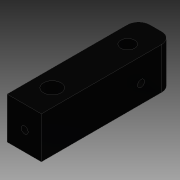
# Autodesk Inventor part: Fixture_Base
Saved by Autodesk Inventor 2015 SP1 (Build 190203100, 203)
## iProperties
Created: 2014-12-16
Part Number: Fixture_Base
Material: Generic
Document SubType Name: Modeling
Designer: amarschn
Density: 1 g/cm^3
Appearance: Anodized - Black
Author: amarschn
Autodesk Inventor part; units mm, degrees
ref_plane "YZ Plane" through (0, 0, 0) normal (1, 0, 0) x (0, 1, 0)
ref_plane "XZ Plane" through (0, 0, 0) normal (0, 1, 0) x (-1, 0, 0)
ref_plane "XY Plane" through (0, 0, 0) normal (0, 0, 1) x (1, 0, 0)
sketch "Sketch1" plane through (0, 0, 0) normal (0, 1, 0) x (-1, 0, 0)
  line L0 (-5.3975, -59.69) -> (5.3975, -59.69)
  line L1 (15.5575, -49.53) -> (15.5575, 59.69)
  line L2 (15.5575, 59.69) -> (-15.5575, 59.69)
  line L3 (-15.5575, 59.69) -> (-15.5575, -49.53)
  line L4 (-15.5575, -59.69) -> (15.5575, 59.69) construction
  line L5 (15.5575, -59.69) -> (-15.5575, 59.69) construction
  arc A0 (5.3975, -59.69) -> (15.5575, -49.53) centre (5.3975, -49.53) ccw
  arc A1 (-15.5575, -49.53) -> (-5.3975, -59.69) centre (-5.3975, -49.53) ccw
  circle A2 centre (0, 34.29) radius 7.9375
  point P0 (0, 0)
  dimension "d0" = 119.38
  dimension "d1" = 31.115
  dimension "d2" = 10.16
  dimension "d3" = 15.875
  dimension "d4" = 25.4
  constraints: 12 end point, 4 point on circle, 4 point on line, 4 tangent, 3 centre point, 2 midpoint, 2 parallel, 1 equal radius, 1 horizontal, 1 perpendicular
  measures "d0" distance of L5.start L1.end
  measures "d1" distance of L1.end L2.end
  measures "d2" radius of A0
  measures "d3" diameter of A2
  measures "d4" distance from line of L2 A2.centre
extrude "Extrusion1" add sketch "Sketch1" along normal blind 37.719
sketch "Sketch2" plane through (0, 37.719, 0) normal (0, 1, 0) x (1, 0, 0)
  line L0 (5.3975, 59.69) -> (-5.3975, 59.69) projected
  point P0 (0, 0)
  point P1 (0, 34.29)
  dimension "d7" = 25.4
  measures "d7" distance from line of point (0, 34.29) L0
hole "Hole1" at (0, 37.719, -34.29) direction (0, -1, 0) diameter 12.7 end through all
hole "Hole3" at (0.3897, 17.4911, 59.69) direction (0, 0, -1) diameter 6.35 depth 12.7 tip angle 118
hole "Hole4" at (-15.5575, 17.5708, -16.4401) direction (1, 0, 0) diameter 6.35 depth 12.7 tip angle 118
hole "Hole5" at (15.5575, 16.4302, -30.8144) direction (-1, 0, 0) diameter 6.35 depth 12.7 tip angle 118
body "Solid1"
